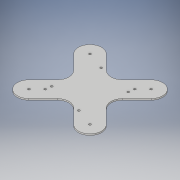
# Autodesk Inventor part: platform 1
Saved by Autodesk Inventor 2019 (Build 230136000, 136)
## iProperties
Created: 2019-02-10
Part Number: platform 1
Material: Generic
Document SubType Name: Modeling
Designer: mashimaro
Density: 1 g/cm^3
Appearance: Default
Author: mashimaro
Autodesk Inventor part; units mm, degrees
ref_plane "YZ Plane" through (0, 0, 0) normal (1, 0, 0) x (0, 1, 0)
ref_plane "XZ Plane" through (0, 0, 0) normal (0, 1, 0) x (-1, 0, 0)
ref_plane "XY Plane" through (0, 0, 0) normal (0, 0, 1) x (1, 0, 0)
sketch "Sketch1" plane through (0, 0, 0) normal (0, 1, 0) x (-1, 0, 0)
  arc A0 (-53.7401, -31.1127) -> (-31.1127, -53.7401) centre (-42.4264, -42.4264) ccw
  arc A1 (31.1127, -53.7401) -> (53.7401, -31.1127) centre (42.4264, -42.4264) ccw
  arc A2 (53.7401, 31.1127) -> (31.1127, 53.7401) centre (42.4264, 42.4264) ccw
  arc A3 (-31.1127, 53.7401) -> (-53.7401, 31.1127) centre (-42.4264, 42.4264) ccw
  line L0 (-53.7401, 31.1127) -> (-33.9411, 11.3137)
  line L1 (11.3137, -33.9411) -> (31.1127, -53.7401)
  line L2 (-53.7401, -31.1127) -> (-33.9411, -11.3137)
  line L3 (11.3137, 33.9411) -> (31.1127, 53.7401)
  line L4 (-31.1127, 53.7401) -> (-11.3137, 33.9411)
  line L5 (33.9411, -11.3137) -> (53.7401, -31.1127)
  line L6 (-31.1127, -53.7401) -> (-11.3137, -33.9411)
  line L7 (33.9411, 11.3137) -> (53.7401, 31.1127)
  arc A4 (11.3137, -33.9411) -> (-11.3137, -33.9411) centre (0, -45.2548) ccw
  arc A5 (33.9411, 11.3137) -> (33.9411, -11.3137) centre (45.2548, 0) ccw
  arc A6 (-11.3137, 33.9411) -> (11.3137, 33.9411) centre (0, 45.2548) ccw
  arc A7 (-33.9411, -11.3137) -> (-33.9411, 11.3137) centre (-45.2548, 0) ccw
  arc A8 (-53.7401, -31.1127) -> (-31.1127, -53.7401) centre (-42.4264, -42.4264) ccw
  arc A9 (31.1127, -53.7401) -> (53.7401, -31.1127) centre (42.4264, -42.4264) ccw
  arc A10 (53.7401, 31.1127) -> (31.1127, 53.7401) centre (42.4264, 42.4264) ccw
  arc A11 (-31.1127, 53.7401) -> (-53.7401, 31.1127) centre (-42.4264, 42.4264) ccw
  line L8 (-53.7401, 31.1127) -> (-33.9411, 11.3137)
  line L9 (11.3137, -33.9411) -> (31.1127, -53.7401)
  line L10 (-53.7401, -31.1127) -> (-33.9411, -11.3137)
  line L11 (11.3137, 33.9411) -> (31.1127, 53.7401)
  line L12 (-31.1127, 53.7401) -> (-11.3137, 33.9411)
  line L13 (33.9411, -11.3137) -> (53.7401, -31.1127)
  line L14 (-31.1127, -53.7401) -> (-11.3137, -33.9411)
  line L15 (33.9411, 11.3137) -> (53.7401, 31.1127)
  arc A12 (11.3137, -33.9411) -> (-11.3137, -33.9411) centre (0, -45.2548) ccw
  arc A13 (33.9411, 11.3137) -> (33.9411, -11.3137) centre (45.2548, 0) ccw
  arc A14 (-11.3137, 33.9411) -> (11.3137, 33.9411) centre (0, 45.2548) ccw
  arc A15 (-33.9411, -11.3137) -> (-33.9411, 11.3137) centre (-45.2548, 0) ccw
  arc A16 (-53.7401, -31.1127) -> (-31.1127, -53.7401) centre (-42.4264, -42.4264) ccw
  arc A17 (31.1127, -53.7401) -> (53.7401, -31.1127) centre (42.4264, -42.4264) ccw
  arc A18 (53.7401, 31.1127) -> (31.1127, 53.7401) centre (42.4264, 42.4264) ccw
  arc A19 (-31.1127, 53.7401) -> (-53.7401, 31.1127) centre (-42.4264, 42.4264) ccw
  line L16 (-53.7401, 31.1127) -> (-33.9411, 11.3137)
  line L17 (11.3137, -33.9411) -> (31.1127, -53.7401)
  line L18 (-53.7401, -31.1127) -> (-33.9411, -11.3137)
  line L19 (11.3137, 33.9411) -> (31.1127, 53.7401)
  line L20 (-31.1127, 53.7401) -> (-11.3137, 33.9411)
  line L21 (33.9411, -11.3137) -> (53.7401, -31.1127)
  line L22 (-31.1127, -53.7401) -> (-11.3137, -33.9411)
  line L23 (33.9411, 11.3137) -> (53.7401, 31.1127)
  arc A20 (11.3137, -33.9411) -> (-11.3137, -33.9411) centre (0, -45.2548) ccw
  arc A21 (33.9411, 11.3137) -> (33.9411, -11.3137) centre (45.2548, 0) ccw
  arc A22 (-11.3137, 33.9411) -> (11.3137, 33.9411) centre (0, 45.2548) ccw
  arc A23 (-33.9411, -11.3137) -> (-33.9411, 11.3137) centre (-45.2548, 0) ccw
  point P0 (0, 0)
  point P1 (0, 0)
  point P2 (0, 0)
  point P3 (0, 0)
  point P4 (0, 0)
  point P5 (0, 0)
  point P6 (0, 0)
  constraints: 48 end point, 48 point on circle, 42 tangent, 24 centre point, 12 coincident, 9 equal radius
extrude "Extrusion1" add sketch "Sketch1" along normal blind 2
sketch "Sketch3" plane through (0, 2, 0) normal (0, 1, 0) x (1, 0, 0)
  arc A0 (53.7401, 31.1127) -> (31.1127, 53.7401) centre (42.4264, 42.4264) ccw projected
  circle A1 centre (42.4264, 42.4264) radius 1.5
  arc A2 (-31.1127, 53.7401) -> (-53.7401, 31.1127) centre (-42.4264, 42.4264) ccw projected
  circle A3 centre (-42.4264, 42.4264) radius 1.5
  arc A4 (-53.7401, -31.1127) -> (-31.1127, -53.7401) centre (-42.4264, -42.4264) ccw projected
  circle A5 centre (-42.4264, -42.4264) radius 1.5
  arc A6 (31.1127, -53.7401) -> (53.7401, -31.1127) centre (42.4264, -42.4264) ccw projected
  circle A7 centre (42.4264, -42.4264) radius 1.5
  circle A8 centre (-31.1127, -31.1127) radius 1.5
  circle A9 centre (31.1127, 31.1127) radius 1.5
  circle A10 centre (-29.9941, -23.2724) radius 1.5
  circle A11 centre (-17.9352, 33.4601) radius 1.5
  circle A12 centre (29.9941, 23.2724) radius 1.5
  circle A13 centre (17.9352, -33.4601) radius 1.5
  point P0 (0, 0)
  dimension "d5" = 3
  dimension "d6" = 3
  dimension "d7" = 3
  dimension "d8" = 3
  dimension "d43" = 3
  dimension "d44" = 3
  dimension "d47" = 3
  dimension "d48" = 3
  dimension "d49" = 3
  dimension "d50" = 3
  constraints: 10 centre point, 4 coincident
  measures "d5" diameter of A1
  measures "d6" diameter of A3
  measures "d7" diameter of A5
  measures "d8" diameter of A7
  measures "d43" diameter of A8
  measures "d44" diameter of A9
  measures "d47" diameter of A10
  measures "d48" diameter of A11
  measures "d49" diameter of A12
  measures "d50" diameter of A13
extrude "Extrusion3" cut sketch "Sketch3" against normal blind 20
body "Solid1"
